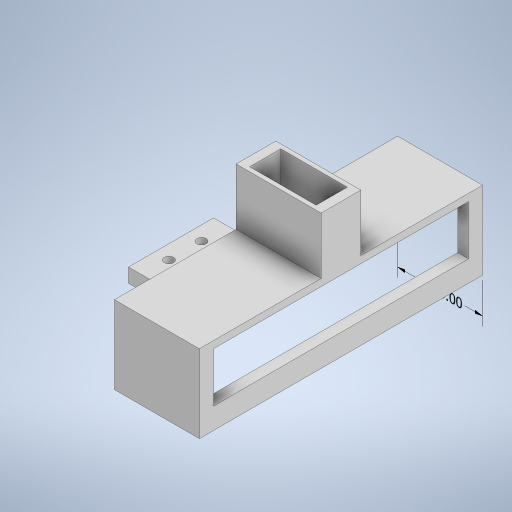
# Autodesk Inventor part: depth_camera_support
Saved by Autodesk Inventor 2023 (Build 270158000, 158)
## iProperties
Created: 2023-05-27
Part Number: depth_camera_support
Material: Genérico
Document SubType Name: Modeling
Designer: inigo
Density: 1 g/cm^3
Appearance: Valor por defecto
Author: inigo
Autodesk Inventor part; units mm, degrees
ref_plane "YZ Plane" through (0, 0, 0) normal (1, 0, 0) x (0, 1, 0)
ref_plane "XZ Plane" through (0, 0, 0) normal (0, 1, 0) x (-1, 0, 0)
ref_plane "XY Plane" through (0, 0, 0) normal (0, 0, 1) x (1, 0, 0)
sketch "Boceto2" plane through (0, 0, 0) normal (0, 1, 0) x (-1, 0, 0)
  line L0 (-30, 100) -> (30, 100)
  line L1 (30, 100) -> (30, -100)
  line L2 (30, -100) -> (-30, -100)
  line L3 (-30, -100) -> (-30, 100)
  line L4 (-30, 100) -> (30, -100) construction
  line L5 (30, 100) -> (-30, -100) construction
  point P0 (0, 0)
  dimension "d0" = 60
  dimension "d1" = 200
  constraints: 12 end point, 2 midpoint, 2 parallel, 1 horizontal, 1 perpendicular
  measures "d0" distance of L1.end L2.end
  measures "d1" distance of L0.end L1.end
extrude "Extrusión1" add sketch "Boceto2" along normal blind 55
sketch "Boceto3" plane through (30, 0, -100) normal (0, 0, -1) x (-1, 0, 0)
  line L0 (7.5, 50) -> (52.5, 50)
  line L1 (52.5, 50) -> (52.5, 0)
  line L2 (52.5, 0) -> (7.5, 0)
  line L3 (7.5, 0) -> (7.5, 50)
  line L4 (0, 0) -> (60, 0) projected
  point P0 (30, 0)
  dimension "d4" = 45
  dimension "d5" = 50
  dimension "d6" = 0
  constraints: 8 end point, 2 parallel, 1 horizontal, 1 perpendicular
  measures "d4" distance of L1.end L2.end
  measures "d5" distance of L0.end L1.end
  measures "d6" distance between parallel lines of L4 L2
extrude "Extrusión2" cut sketch "Boceto3" against normal blind 190
sketch "Boceto4" plane through (30, 0, 100) normal (1, 0, 0) x (0, 0, -1)
  line L0 (10, 50) -> (10, 0) projected
  line L1 (10, 50) -> (10, 0)
  line L2 (200, 0) -> (0, 0) projected
  line L3 (10, 50) -> (10, 0)
  line L4 (190, 0) -> (190, 50)
  line L5 (200, 50) -> (10, 50) projected
  line L6 (200, 0) -> (200, 55) projected
  line L7 (10, 15) -> (190, 15)
  line L8 (10, 50) -> (190, 50)
  point P0 (100, 0)
  point P1 (200, 27.5)
  dimension "d9" = 10
  dimension "d10" = 15
  constraints: 10 end point, 5 point on line, 3 perpendicular, 2 vertical, 1 midpoint
  measures "d9" distance from line of point (200, 27.5) L4
  measures "d10" distance between parallel lines of L2 L7
extrude "Extrusión3" cut sketch "Boceto4" against normal blind 10 contours L5 L4 L7 L0
sketch "Boceto5" plane through (0, 0, 0) normal (0, 1, 0) x (-1, 0, 0)
  line L0 (30, -100) -> (30, 100) projected
  line L1 (30, 0) -> (60, 0)
  line L2 (90, 30) -> (30, 30)
  line L3 (30, 30) -> (30, -30)
  line L4 (30, -30) -> (90, -30)
  line L5 (90, -30) -> (90, 30)
  line L6 (90, 30) -> (30, -30) construction
  line L7 (30, 30) -> (90, -30) construction
  circle A0 centre (50, 11.5) radius 3.25
  circle A1 centre (50, -11.5) radius 3.25
  circle A2 centre (80, 11.5) radius 3.25
  circle A3 centre (80, -11.5) radius 3.25
  point P0 (0, 0)
  dimension "d16" = 30
  dimension "d17" = 60
  dimension "d18" = 60
  dimension "d19" = 6.5
  dimension "d20" = 20
  dimension "d21" = 18.5
  dimension "d22" = 23
  dimension "d23" = 6.5
  dimension "d24" = 30
  dimension "d25" = 18.5
  constraints: 14 end point, 4 centre point, 3 midpoint, 2 horizontal, 2 parallel, 2 symmetric about line, 1 perpendicular, 2 other
  measures "d16" distance of L1.start L1.end
  measures "d17" distance of L4.end L3.end
  measures "d18" distance of L3.end L2.end
  measures "d19" diameter of A0
  measures "d20" distance from line of L0 A0.centre
  measures "d21" distance from line of L2 A0.centre
  measures "d22" distance of A1.centre A0.centre
  measures "d23" diameter of A2
  measures "d24" distance of A0.centre A2.centre
  measures "d25" distance from line of L2 A2.centre
extrude "Extrusión4" add sketch "Boceto5" along normal blind 10
sketch "Boceto6" plane through (0, 55, 0) normal (0, 1, 0) x (1, 0, 0)
  line L0 (-30, 30) -> (-30, -30) projected
  line L1 (30, -14) -> (-30, -14)
  line L2 (-30, -14) -> (-30, 14)
  line L3 (-30, 14) -> (30, 14)
  line L4 (30, 14) -> (30, -14)
  line L5 (30, -14) -> (-30, 14) construction
  line L6 (-30, -14) -> (30, 14) construction
  point P0 (0, 0)
  dimension "d28" = 28
  constraints: 12 end point, 2 midpoint, 2 parallel, 1 horizontal, 1 perpendicular, 1 point on line
  measures "d28" distance of L1.end L2.end
extrude "Extrusión5" add sketch "Boceto6" along normal blind 40
sketch "Boceto7" plane through (0, 95, 0) normal (0, 1, 0) x (1, 0, 0)
  line L0 (-23.5, 11) -> (23.5, 11)
  line L1 (23.5, 11) -> (23.5, -11)
  line L2 (23.5, -11) -> (-23.5, -11)
  line L3 (-23.5, -11) -> (-23.5, 11)
  line L4 (-23.5, 11) -> (23.5, -11) construction
  line L5 (23.5, 11) -> (-23.5, -11) construction
  point P0 (0, 0)
  dimension "d31" = 47
  dimension "d32" = 22
  constraints: 12 end point, 2 midpoint, 2 parallel, 1 horizontal, 1 perpendicular
  measures "d31" distance of L1.end L2.end
  measures "d32" distance of L0.end L1.end
extrude "Extrusión6" cut sketch "Boceto7" against normal blind 43
sketch "Boceto8" plane through (-30, 0, 100) normal (-1, 0, 0) x (0, 0, 1)
  line L0 (-200, 55) -> (-114, 55) projected
  line L1 (0, 55) -> (-86, 55) projected
  line L2 (-114, 55) -> (-86, 55)
  line L3 (-111, 65) -> (-89, 65)
  line L4 (-89, 65) -> (-89, 55)
  line L5 (-89, 55) -> (-111, 55)
  line L6 (-111, 55) -> (-111, 65)
  line L7 (-111, 65) -> (-89, 55) construction
  line L8 (-89, 65) -> (-111, 55) construction
  point P0 (-100, 0)
  point P1 (-100, 60)
  dimension "d35" = 22
  dimension "d36" = 10
  dimension "d37" = 0
  constraints: 14 end point, 2 midpoint, 2 parallel, 1 collinear, 1 horizontal, 1 perpendicular
  measures "d35" distance of L4.end L5.end
  measures "d36" distance of L3.end L4.end
  measures "d37" distance between parallel lines of L5 L2
extrude "Extrusión7" cut sketch "Boceto8" against normal blind 10
ref_plane "Plano de trabajo1" through (30, 55, 0) normal (0, 0, -1) x (-1, 0, 0)
sketch "Boceto10" plane through (30, 55, 0) normal (0, 0, -1) x (-1, 0, 0)
  line L0 (60.12, -45) -> (60.12, 17.4198)
  line L1 (60.12, -45) -> (60.12, 13.5667)
  line L2 (60.12, -45) -> (137.1989, -45)
  line L3 (60.12, -19.9519) -> (80.5233, -61.6073)
  line L4 (120, -45) -> (60, -45) projected
  point P0 (30, -55)
  point P1 (72.3889, -45)
  dimension "d41" = 0
  constraints: 8 end point, 2 point on line
  measures "d41" distance between parallel lines of L4 L2
extrude "Extrusión8" add sketch "Boceto10" along normal mid plane 15
